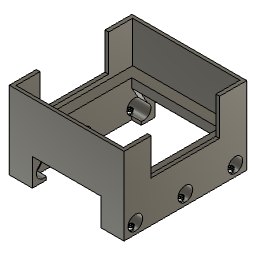
Camera Cradle Version 1 v4 (Autodesk Fusion 360 design; units mm, degrees)
Autodesk Fusion 360 part; units mm, degrees
sketch "Sketch1" plane through (0, 0, 0) normal (0, 0, 1) x (1, 0, 0)
  line L0 (23.5, -25.5) -> (-23.5, -25.5)
  line L1 (-23.5, -25.5) -> (-23.5, 25.5)
  line L2 (-23.5, 25.5) -> (23.5, 25.5)
  line L3 (23.5, 25.5) -> (23.5, -25.5)
  line L4 (23.5, -25.5) -> (-23.5, 25.5) construction
  line L5 (-23.5, -25.5) -> (23.5, 25.5) construction
  line L6 (25.0981, -26.8493) -> (-25.0981, -26.8493)
  line L7 (-25.0981, -26.8493) -> (-25.0981, 26.8493)
  line L8 (-25.0981, 26.8493) -> (25.0981, 26.8493)
  line L9 (25.0981, 26.8493) -> (25.0981, -26.8493)
  line L10 (25.0981, -26.8493) -> (-25.0981, 26.8493) construction
  line L11 (-25.0981, -26.8493) -> (25.0981, 26.8493) construction
  line L12 (19.1358, -20.7643) -> (-19.1358, -20.7643)
  line L13 (-19.1358, -20.7643) -> (-19.1358, 20.7643)
  line L14 (-19.1358, 20.7643) -> (19.1358, 20.7643)
  line L15 (19.1358, 20.7643) -> (19.1358, -20.7643)
  line L16 (19.1358, -20.7643) -> (-19.1358, 20.7643) construction
  line L17 (-19.1358, -20.7643) -> (19.1358, 20.7643) construction
  dimension "d1" = 47
  dimension "d2" = 51
  constraint horizontal L0
  constraint perpendicular L0 L1
  constraint parallel L0 L2
  constraint parallel L1 L3
  constraint coincident L4 origin
  constraint coincident L5 origin
  constraint horizontal L6
  constraint perpendicular L6 L7
  constraint parallel L6 L8
  constraint parallel L7 L9
  constraint coincident L10 origin
  constraint coincident L11 origin
  constraint horizontal L12
  constraint perpendicular L12 L13
  constraint parallel L12 L14
  constraint parallel L13 L15
  constraint coincident L4 L12.start
  constraint coincident L16 origin
  constraint coincident L17 origin
  measures "d1" distance of L1.end L2.end
  measures "d2" distance of L0.end L1.end
sketch "Sketch2" plane through (0, 0, 0) normal (1, 0, 0) x (0, 1, 0)
  line L0 (-15, 1.9999) -> (15, 1.9999)
  line L1 (15, 1.9999) -> (15, 15)
  line L2 (15, 15) -> (-15, 15)
  line L3 (-15, 15) -> (-15, 1.9999)
  constraint perpendicular L0 L1
  constraint parallel L0 L2
  constraint parallel L1 L3
  constraint horizontal L0
extrude "Extrude1" add sketch "Sketch1" against normal blind 5 contours L0 L1 L2 L3 | L6 L7 L8 L9 makes body 1
extrude "Extrude2" add sketch "Sketch1" along normal blind 10 separate body contours L6 L7 L8 L9 makes body 2
extrude "Extrude3" cut sketch "Sketch2" along normal mid plane 120 bodies 2
extrude "Extrude4" add 1 faces at (6.3786, -24.821, -5) along direction (0, 0, -1) blind 4 on bodies 1 bodies 1
sketch "Sketch4" plane through (25.0981, 0, 0) normal (1, 0, 0) x (0, 1, 0)
  line L0 (26.8493, 0) -> (-26.8493, 0)
  line L1 (-26.8493, 0) -> (-26.8493, -9)
  line L2 (-26.8493, -9) -> (26.8493, -9)
  line L3 (26.8493, -9) -> (26.8493, 0)
  line L4 (0, 0) -> (0, -4.5)
  line L5 (0, -4.5) -> (21.875, -4.5)
  line L6 (0, -4.5) -> (-21.875, -4.5)
  dimension "d12" = 21.875
  dimension "d13" = 21.875
  constraint coincident L4.start origin
  constraint perpendicular L2 L4
  constraint perpendicular L4 L5
  constraint perpendicular L4 L6
  measures "d12" distance of L4.end L5.end
  measures "d13" distance of L4.end L6.end
hole "Hole1" at (25.0981, -21.875, -4.5) at (25.0981, 0, -4.5) at (25.0981, 21.875, -4.5) direction (-1, 0, 0) diameter 6.4 depth 60.4 tip angle 118 bodies 1
sketch "Sketch5" plane through (0, 0, -9) normal (0, 0, -1) x (1, 0, 0)
  line L0 (19.1358, -20.7643) -> (-19.1358, -20.7643)
  line L1 (-19.1358, -20.7643) -> (-19.1358, 20.7643)
  line L2 (-19.1358, 20.7643) -> (19.1358, 20.7643)
  line L3 (19.1358, 20.7643) -> (19.1358, -20.7643)
  line L4 (-25.0981, -26.8493) -> (25.0981, -26.8493)
  line L5 (25.0981, -26.8493) -> (25.0981, 26.8493)
  line L6 (25.0981, 26.8493) -> (-25.0981, 26.8493)
  line L7 (-25.0981, 26.8493) -> (-25.0981, -26.8493)
  line L8 (22.1169, 0) -> (25.0981, 0)
  line L9 (22.1169, 0) -> (22.1169, -21.875)
  line L10 (22.1169, 0) -> (22.1169, 21.875)
  line L11 (-25.0981, 0) -> (-22.1169, 0)
  line L12 (-22.1169, 0) -> (-22.1169, 21.875)
  line L13 (-22.1169, 0) -> (-22.1169, -21.875)
  dimension "d17" = 21.875
  dimension "d18" = 21.875
  dimension "d27" = 21.875
  dimension "d28" = 21.875
  constraint midpoint L5 L8.end
  constraint perpendicular L8 L9
  constraint perpendicular L8 L10
  constraint midpoint L7 L11.start
  constraint perpendicular L11 L12
  constraint perpendicular L11 L13
  measures "d17" distance of L8.start L9.end
  measures "d18" distance of L8.start L10.end
  measures "d27" distance of L11.end L12.end
  measures "d28" distance of L11.end L13.end
hole "Hole2" at (22.1169, -21.875, -9) at (22.1169, 0, -9) at (22.1169, 21.875, -9) at (-22.1169, -21.875, -9) at (-22.1169, 0, -9) at (-22.1169, 21.875, -9) direction (0, 0, 1) diameter 3.416 depth 4.4 tip angle 118 bodies 1
thread "Thread1" "ANSI Unified Screw Threads 0.164(#8) 8-32 UNC 2B" major diameter 4.1656 minor diameter 3.4163 pitch 0.7937 angle 60 modelled right hand crest width 0.2341 on face at (22.2528, -20.1724, -8.4034) crest through (20.4088, -21.875, -8.8016) on face at (22.2528, 1.7026, -8.4034) crest through (20.4088, 0, -8.8016) on face at (22.2528, 23.5776, -8.4034) crest through (20.4088, 21.875, -8.8016) on face at (-21.981, -20.1724, -8.4034) crest through (-23.8251, -21.875, -8.8016) on face at (-21.981, 1.7026, -8.4034) crest through (-23.8251, 0, -8.8016) on face at (-21.981, 23.5776, -8.4034) crest through (-23.8251, 21.875, -8.8016) on bodies 1
move_body "Move1" bodies 2 to x (1, 0, 0) y (0, 1, 0) z (0, 0, 1) at (0, 0, 7)
extrude "Extrude5" add 1 faces at (6.3786, -24.821, 0) along direction (0, 0, 1) blind 7 on bodies 1 bodies 1 2
extrude "Extrude6" add 2 faces at (-24.5654, 22.4498, 17) (-24.5654, -22.4498, 17) along direction (0, 0, 1) blind 8 on bodies 1 bodies 1
chamfer "Chamfer1" distance 8 angle 45 2 edges at (0, 20.7643, -1.4989) (0, -20.7643, -1.4989) on bodies 1
sketch "Sketch6" plane through (0, 26.8493, 0) normal (0, 1, 0) x (-1, 0, 0)
  line L0 (-25.0981, 25) -> (-25.0981, -9)
  line L1 (-25.0981, -9) -> (25.0981, -9)
  line L2 (25.0981, -9) -> (25.0981, 25)
  line L3 (25.0981, 25) -> (-25.0981, 25)
  line L4 (-14.9998, -9) -> (15, -9)
  line L5 (15, -9) -> (15, 3)
  line L6 (15, 3) -> (-14.9998, 3)
  line L7 (-14.9998, 3) -> (-14.9998, -9)
  constraint horizontal L4
  constraint vertical L5
  constraint horizontal L6
  constraint vertical L7
  constraint coincident L1 L4.start
extrude "Extrude7" cut sketch "Sketch6" against normal blind 82 contours L1 L4 L5 L6 L7 bodies 1
copy_body "Body->Comp1" bodies 1 removing the originals makes body 3 in component "Component"
component "Component" placed x (1, 0, 0) y (0, 1, 0) z (0, 0, 1) at (0, 0, 0)
